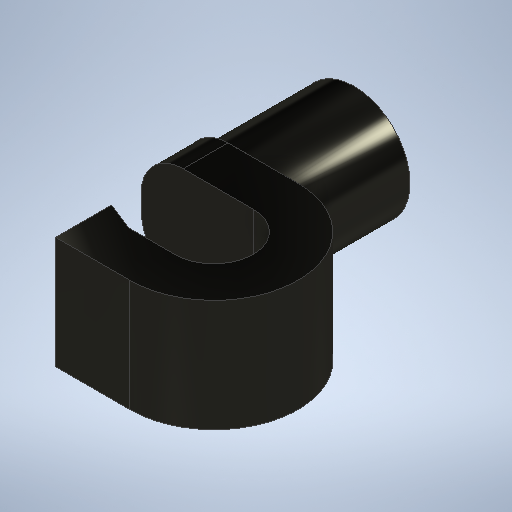
# Autodesk Inventor part: Hitch to the Polar Express [Copy]
Saved by Autodesk Inventor 2025.1 (Build 291241020, 241B)
## iProperties
Created: 2022-11-22
Part Number: Hitch to the Polar Express [Copy]
Material: Generic
Document SubType Name: Modeling
Designer: mc_vlongo24
Density: 1 g/cm^3
Appearance: Default
Author: mc_vlongo24
Autodesk Inventor part; units mm, degrees
ref_plane "YZ Plane" through (0, 0, 0) normal (1, 0, 0) x (0, 1, 0)
ref_plane "XZ Plane" through (0, 0, 0) normal (0, 1, 0) x (-1, 0, 0)
ref_plane "XY Plane" through (0, 0, 0) normal (0, 0, 1) x (1, 0, 0)
sketch "Sketch1" plane through (0, 0, 0) normal (0, 0, 1) x (1, 0, 0)
  line L0 (0, 0) -> (12.7, 0)
  line L1 (12.7, 0) -> (12.7, -12.7)
  line L2 (12.7, -12.7) -> (0, -12.7)
  line L3 (0, -12.7) -> (0, 0)
  point P0 (6.35, -12.7)
  point P1 (6.35, 0)
  dimension "d0" = 12.7
  dimension "d1" = 12.7
  constraints: 8 end point, 2 midpoint, 2 parallel, 1 horizontal, 1 perpendicular
  measures "d0" distance of point (6.35, -12.7) point (6.35, 0)
  measures "d1" distance between parallel lines of L3 L1
extrude "Extrusion1" add sketch "Sketch1" along normal blind 12.7
fillet "Fillet1" radius 6.35 4 edges at (12.7, 0, 6.35) (0, 0, 6.35) (0, -12.7, 6.35) (12.7, -12.7, 6.35)
sketch "Sketch2" plane through (6.35, -6.35, 12.7) normal (0, 0, 1) x (1, 0, 0)
  line L0 (-2.0483, -0.0105) -> (1.7617, -0.0105)
  line L1 (1.7617, -0.0105) -> (1.7617, -0.03)
  line L2 (1.7617, -0.03) -> (-2.0483, -0.03)
  line L3 (-2.0483, -0.03) -> (-2.0483, -0.0105)
  point P0 (-6.35, 6.35)
  constraints: 8 end point, 2 parallel, 1 horizontal, 1 perpendicular
extrude "Extrusion2" add sketch "Sketch2" along normal blind 2.54
sketch "Sketch4" plane through (4.3017, -6.3605, 12.7) normal (0, 1, 0) x (1, 0, 0)
  line L0 (8.3983, 0) -> (-4.3017, 0) projected
  arc A0 (8.3983, -19.05) -> (8.3983, 0) centre (8.3983, -9.525) ccw
  line L1 (8.3983, -19.05) -> (-0.04, -19.05)
  line L2 (-0.04, -19.05) -> (-0.04, -13.97)
  line L3 (-0.04, -13.97) -> (8.3983, -13.97)
  line L4 (-4.3017, 0) -> (-4.3017, -5.08)
  line L5 (-4.3017, -5.08) -> (8.3983, -5.08)
  arc A1 (8.3983, -13.97) -> (8.3983, -5.08) centre (8.3983, -9.525) ccw
  point P0 (-4.3017, 12.7)
  dimension "d10" = 19.05
  dimension "d11" = 5.08
  dimension "d12" = 5.08
  constraints: 10 end point, 4 point on circle, 3 tangent, 2 centre point, 2 parallel, 2 vertical, 1 horizontal
  measures "d10" distance of L0.start L1.start
  measures "d11" distance of L1.end L2.end
  measures "d12" distance of L0.end L4.end
extrude "Extrusion3" add sketch "Sketch4" along normal mid plane 12.7
fillet "Fillet2" radius 6.35 1 edges at (0, -12.7105, 15.24)
fillet "Fillet3" radius 4.7625 1 edges at (0, -0.0105, 15.24)
sketch "Sketch5" plane through (12.7, -0.0105, 26.67) normal (0, 0, -1) x (-1, 0, 0)
  line L0 (0, 0) -> (8.4383, 0) projected
  line L1 (8.4383, -12.7) -> (0, -12.7) projected
  line L2 (8.4383, 0) -> (5.2633, 0)
  line L3 (5.2633, 0) -> (5.2633, -12.7)
  line L4 (5.2633, -12.7) -> (8.4383, -12.7)
  line L5 (8.4383, -12.7) -> (8.4383, 0)
  point P0 (12.7, 0.0105)
  point P1 (5.2633, 0)
  dimension "d17" = 3.175
  constraints: 8 end point, 2 parallel, 1 horizontal, 1 perpendicular, 1 point on line
  measures "d17" distance between parallel lines of L5 L3
extrude "Extrusion4" add sketch "Sketch5" along normal blind 1.27
chamfer "Chamfer1" distance 3.175 angle 21.8 1 edges at (7.4367, -6.3605, 25.4) measured on face at (6.3784, -4.2438, 25.4)
body "Solid1"
